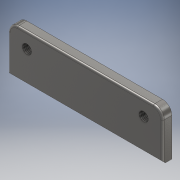
# Autodesk Inventor part: BearingHousing_Jack
Saved by Autodesk Inventor 2018 (Build 220112000, 112)
## iProperties
Created: 2018-02-06
Part Number: BearingHousing_Jack
Material: Steel, Galvanized
Document SubType Name: Modeling
Designer: P136265
Density: 7.85 g/cm^3
Appearance: Galvanized
Author: P136265
Autodesk Inventor part; units mm, degrees
ref_plane "YZ Plane" through (0, 0, 0) normal (1, 0, 0) x (0, 1, 0)
ref_plane "XZ Plane" through (0, 0, 0) normal (0, 1, 0) x (-1, 0, 0)
ref_plane "XY Plane" through (0, 0, 0) normal (0, 0, 1) x (1, 0, 0)
sketch "Sketch1" plane through (0, 0, 0) normal (0, 0, 1) x (1, 0, 0)
  line L0 (-41, -2.5) -> (41, -2.5)
  line L1 (41, -2.5) -> (41, 2.5)
  line L2 (41, 2.5) -> (-41, 2.5)
  line L3 (-41, 2.5) -> (-41, -2.5)
  line L4 (-41, -2.5) -> (41, 2.5) construction
  line L5 (41, -2.5) -> (-41, 2.5) construction
  point P0 (0, 0)
  dimension "d0" = 82
  dimension "d1" = 5
  constraints: 12 end point, 2 midpoint, 2 parallel, 1 horizontal, 1 perpendicular
  measures "d0" distance of L2.end L1.end
  measures "d1" distance of L1.end L0.end
extrude "Extrusion1" add sketch "Sketch1" along normal blind 25
chamfer "Chamfer1" distance 1.5 angle 45 1 edges at (0, -2.5, 0)
fillet "Fillet1" radius 5 2 edges at (-41, 0, 25) (41, 0, 25)
sketch "Sketch2" plane through (-41, 2.5, 0) normal (0, 1, 0) x (1, 0, 0)
  circle A0 centre (10, -17) radius 3 construction
  circle A1 centre (72, -17) radius 3 construction
  line L0 (77, -25) -> (5, -25) construction
  line L1 (0, 0) -> (0, -20) construction
  line L2 (82, 0) -> (82, -20) construction
  point P0 (41, 0)
  dimension "d8" = 6
  dimension "d9" = 6
  dimension "d10" = 8
  dimension "d11" = 10
  dimension "d12" = 10
  dimension "d13" = 8
  constraints: 2 centre point
  measures "d8" diameter of A0
  measures "d9" diameter of A1
  measures "d10" distance from line of L0 A0.centre
  measures "d11" distance from line of L1 A0.centre
  measures "d12" distance from line of L2 A1.centre
  measures "d13" distance from line of L0 A1.centre
hole "Hole1" at (-31, 2.5, 17) at (31, 2.5, 17) direction (0, -1, 0) diameter 5 end through all
thread "Thread1" size "M5x0.8" class "6H" standard "ANSI Metric M Profile" full length
thread "Thread2" size "M5x0.8" class "6H" standard "ANSI Metric M Profile" full length
fillet "Fillet2" radius 1 5 edges at (-39.5355, -2.5, 23.5355) (0, -2.5, 25) (39.5355, -2.5, 23.5355) (41, -2.5, 10.75) (-41, -2.5, 10.75)
body "Solid1"
